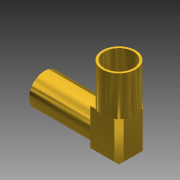
# Autodesk Inventor part: SMA_RightAngle
Saved by Autodesk Inventor 2014 (Build 180170000, 170)
## iProperties
Created: 2015-01-07
Part Number: SMA_RightAngle
Material: Generic
Document SubType Name: Modeling
Designer: Owner
Density: 1 g/cm^3
Appearance: Gold - Metal
Author: Owner
Autodesk Inventor part; units mm, degrees
ref_plane "YZ Plane" through (0, 0, 0) normal (1, 0, 0) x (0, 1, 0)
ref_plane "XZ Plane" through (0, 0, 0) normal (0, 1, 0) x (-1, 0, 0)
ref_plane "XY Plane" through (0, 0, 0) normal (0, 0, 1) x (1, 0, 0)
sketch "Sketch1" plane through (0, 0, 0) normal (0, 1, 0) x (-1, 0, 0)
  line L0 (-3, 1.2097) -> (3, 1.2097)
  line L1 (3, 1.2097) -> (3, -4.7903)
  line L2 (3, -4.7903) -> (-3, -4.7903)
  line L3 (-3, -4.7903) -> (-3, 1.2097)
  point P0 (0, 0)
  dimension "d0" = 6
  dimension "d1" = 6
  constraints: 8 end point, 2 parallel, 1 horizontal, 1 perpendicular
  measures "d0" distance of L0.start L0.end
  measures "d1" distance of L0.end L1.end
extrude "Extrusion1" add sketch "Sketch1" along normal blind 8.7
sketch "Sketch2" plane through (0, 8.7, 0) normal (0, 1, 0) x (1, 0, 0)
  circle A0 centre (0, 1.7903) radius 3.5
  point P0 (0, 0)
  dimension "d4" = 7
  constraints: 1 centre point
  measures "d4" diameter of A0
extrude "Extrusion2" add sketch "Sketch2" along normal blind 8.4
sketch "Sketch3" plane through (0, 17.1, -1.7903) normal (0, 1, 0) x (1, 0, 0)
  circle A0 centre (0, 0) radius 3.5 projected
  circle A1 centre (0, 0) radius 3.05
  point P0 (0, -1.7903)
  dimension "d7" = 6.1
  constraints: 1 centre point, 1 coincident
  measures "d7" diameter of A1
extrude "Extrusion3" cut sketch "Sketch3" against normal blind 8 contours A1
sketch "Sketch4" plane through (-3, 0, -4.7903) normal (-1, 0, 0) x (0, 0, 1)
  circle A0 centre (3, 4) radius 3.24
  line L0 (6.5, 17.1) -> (-0.5, 17.1) projected
  point P0 (4.7903, 0)
  dimension "d10" = 6.48
  dimension "d11" = 13.1
  constraints: 1 centre point
  measures "d10" diameter of A0
  measures "d11" distance from line of A0.centre L0
extrude "Extrusion4" add sketch "Sketch4" along normal blind 12.7
chamfer "Chamfer1" distance 1 angle 45 5 edges at (3, 4.35, 1.2097) (3, 4.35, -4.7903) (3, 0, -1.7903) (0, 0, 1.2097) (0, 0, -4.7903)
body "Solid1"
